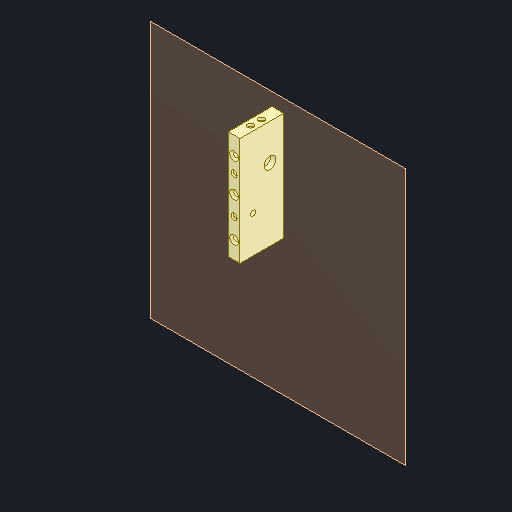
# Autodesk Inventor part: middle_gear_holder
Saved by Autodesk Inventor 2023 (Build 270158000, 158)
## iProperties
Created: 2024-04-23
Part Number: middle_gear_holder
Material: Nylon 6/6
Document SubType Name: Modeling
Designer: szymo
Density: 1.13 g/cm^3
Appearance: Nylon 6
Mass: 25.6721 g
Surface Area: 95.1123 cm^2
Volume: 22.7187 cm^3
Author: szymo
Autodesk Inventor part; units mm, degrees
ref_plane "YZ Plane" through (0, 0, 0) normal (1, 0, 0) x (0, 1, 0)
ref_plane "XZ Plane" through (0, 0, 0) normal (0, 1, 0) x (-1, 0, 0)
ref_plane "Work Plane1" through (0, 0, 0) normal (0, 0, 1) x (1, 0, 0)
ref_plane "Work Plane2" through (-89, -40.3889, 33.5) normal (0, 0, 1) x (1, 0, 0)
sketch "Sketch1" plane through (0, 0, 0) normal (0, 0, 1) x (1, 0, 0)
  line L0 (23.5, 88.5) -> (-23.5, 88.5) projected
  line L1 (-23.5, 88.5) -> (-23.5, 36.5) projected
  line L2 (-26.5, 33.5) -> (-89, 33.5) projected
  line L3 (-89, 33.5) -> (-89, -72.5) projected
  line L4 (-89, -72.5) -> (-77, -72.5) projected
  line L5 (-74, -75.5) -> (-74, -93.5) projected
  line L6 (-74, -93.5) -> (74, -93.5) projected
  line L7 (74, -93.5) -> (74, -75.5) projected
  line L8 (77, -72.5) -> (89, -72.5) projected
  line L9 (89, -72.5) -> (89, 33.5) projected
  line L10 (89, 33.5) -> (26.5, 33.5) projected
  line L11 (23.5, 36.5) -> (23.5, 88.5) projected
  line L12 (-4.5, 81.5) -> (-4.5, 36.5) projected
  line L13 (-7.5, 33.5) -> (-13.5, 33.5) projected
  line L14 (-16.5, 36.5) -> (-16.5, 81.5) projected
  line L15 (7.5, 84.5) -> (13.5, 84.5) projected
  line L16 (16.5, 81.5) -> (16.5, 36.5) projected
  line L17 (13.5, 33.5) -> (7.5, 33.5) projected
  line L18 (4.5, 36.5) -> (4.5, 81.5) projected
  line L19 (-13.5, 84.5) -> (-7.5, 84.5) projected
  line L20 (-4.5, 88.5) -> (4.5, 88.5)
  line L21 (4.5, 88.5) -> (4.5, 5.75)
  line L22 (4.5, 5.75) -> (-4.5, 5.75)
  line L23 (-4.5, 5.75) -> (-4.5, 88.5)
  line L24 (-32.2, 4.75) -> (-59.9, 4.75)
  arc A0 (13.5, 33.5) -> (16.5, 36.5) centre (13.5, 36.5) ccw projected
  arc A1 (4.5, 36.5) -> (7.5, 33.5) centre (7.5, 36.5) ccw projected
  arc A2 (7.5, 84.5) -> (4.5, 81.5) centre (7.5, 81.5) ccw projected
  arc A3 (16.5, 81.5) -> (13.5, 84.5) centre (13.5, 81.5) ccw projected
  arc A4 (-4.5, 81.5) -> (-7.5, 84.5) centre (-7.5, 81.5) ccw projected
  arc A5 (-7.5, 33.5) -> (-4.5, 36.5) centre (-7.5, 36.5) ccw projected
  arc A6 (-16.5, 36.5) -> (-13.5, 33.5) centre (-13.5, 36.5) ccw projected
  arc A7 (-13.5, 84.5) -> (-16.5, 81.5) centre (-13.5, 81.5) ccw projected
  arc A8 (-26.5, 33.5) -> (-23.5, 36.5) centre (-26.5, 36.5) ccw projected
  arc A9 (-74, -75.5) -> (-77, -72.5) centre (-77, -75.5) ccw projected
  arc A10 (77, -72.5) -> (74, -75.5) centre (77, -75.5) ccw projected
  arc A11 (23.5, 36.5) -> (26.5, 33.5) centre (26.5, 36.5) ccw projected
  circle A12 centre (21.5, -85.5) radius 1.8 projected
  circle A13 centre (-64.5, -85.5) radius 1.8 projected
  circle A14 centre (83.4, -16.3889) radius 1.8 projected
  circle A15 centre (-83.4, -19.2889) radius 1.8 projected
  circle A16 centre (-21.5, -85.5) radius 1.8 projected
  circle A17 centre (64.5, -85.5) radius 1.8 projected
  circle A18 centre (39.125, 4.3375) radius 1.0065 projected
  circle A19 centre (-72.95, 4.275) radius 1.0065 projected
  circle A20 centre (39.125, 25.9125) radius 1.0065 projected
  circle A21 centre (72.95, 12.275) radius 1.0065 projected
  circle A22 centre (86, 30.5) radius 1.0065 projected
  circle A23 centre (-86, 30.5) radius 1.0065 projected
  circle A24 centre (-39.125, 12.3375) radius 1.0065 projected
  circle A25 centre (-72.95, 25.975) radius 1.0065 projected
  circle A26 centre (-72.95, 12.275) radius 1.0065 projected
  circle A27 centre (-39.125, 25.9125) radius 1.0065 projected
  circle A28 centre (-86, 7.75) radius 1.0065 projected
  circle A29 centre (86, 7.75) radius 1.0065 projected
  circle A30 centre (72.95, 25.975) radius 1.0065 projected
  circle A31 centre (39.125, 12.3375) radius 1.0065 projected
  circle A32 centre (-39.125, 4.3375) radius 1.0065 projected
  circle A33 centre (72.95, 4.275) radius 1.0065 projected
  circle A34 centre (78, -67.1725) radius 1.2295 projected
  circle A35 centre (-24.1, -73.1) radius 1.2295 projected
  circle A36 centre (24.1, -24.9) radius 1.2295 projected
  circle A37 centre (-42.4984, -44.6666) radius 1.2295 projected
  circle A38 centre (-79, -42.3889) radius 1.2295 projected
  circle A39 centre (-19.5, 28.875) radius 1.2295 projected
  circle A40 centre (19.5, 9.55) radius 1.2295 projected
  circle A41 centre (19.5, 47.3) radius 1.2295 projected
  circle A42 centre (-19.5, 47.3) radius 1.2295 projected
  circle A43 centre (0, 74.7) radius 1.2295 projected
  circle A44 centre (-19.4231, 74.8077) radius 1.2295 projected
  circle A45 centre (19.5, 74.7) radius 1.2295 projected
  circle A46 centre (0, 49.05) radius 1.2295 projected
  circle A47 centre (19.5, 28.875) radius 1.2295 projected
  circle A48 centre (0, 19.125) radius 1.2295 projected
  circle A49 centre (-19.5, 9.55) radius 1.2295 projected
  circle A50 centre (-78, -67.1725) radius 1.2295 projected
  circle A51 centre (-24.1, -24.9) radius 1.2295 projected
  circle A52 centre (24.1, -73.1) radius 1.2295 projected
  circle A53 centre (42.5, -44.6649) radius 1.2295 projected
  circle A54 centre (79, -42.3889) radius 1.2295 projected
  line L25 (74, -12.9454) -> (74, -38.6649) projected
  line L26 (32.5736, -41.3399) -> (10.2484, -66.6122) projected
  line L27 (40.7223, -24.1882) -> (40.7223, -2.7315) projected
  line L28 (15.0791, 0.2685) -> (31.7223, 0.2685) projected
  line L29 (-68.7516, -10.9592) -> (-46.0313, -36.6788) projected
  line L30 (-74, -38.6649) -> (-74, -12.9454) projected
  line L31 (43.7223, 0.2685) -> (62.6769, 0.2685) projected
  line L32 (-40.7223, -2.7315) -> (-40.7223, -24.1882) projected
  line L33 (-45.9707, -26.1743) -> (-64.9252, -4.7177) projected
  line L34 (46.0313, -36.6788) -> (68.7516, -10.9592) projected
  line L35 (-62.6769, 0.2685) -> (-43.7223, 0.2685) projected
  line L36 (34.7223, -2.7315) -> (34.7223, -24.9078) projected
  line L37 (29.5555, -26.9826) -> (10.5667, -7.1519) projected
  line L38 (-31.598, -53.0174) -> (-25.9833, -59.3733) projected
  line L39 (-10.5667, -7.1519) -> (-29.5555, -26.9826) projected
  line L40 (-34.7223, -24.9078) -> (-34.7223, -2.7315) projected
  line L41 (-31.7223, 0.2685) -> (-15.0791, 0.2685) projected
  line L42 (25.9833, -59.3733) -> (31.598, -53.0174) projected
  line L43 (64.9252, -4.7177) -> (45.9707, -26.1743) projected
  line L44 (-10.2484, -66.6122) -> (-32.5736, -41.3399) projected
  line L45 (-32.4921, -37.2789) -> (-10.1668, -13.9638) projected
  line L46 (10.1668, -13.9638) -> (32.4921, -37.2789) projected
  line L47 (29.5955, -81.1563) -> (25.3044, -62.0157) projected
  arc A55 (25.9833, -59.3733) -> (25.3044, -62.0157) centre (28.2317, -61.3594) ccw projected
  line L48 (43.9754, -47.6649) -> (68.9203, -47.6649) projected
  arc A56 (71.5475, -52.1134) -> (68.9203, -47.6649) centre (68.9203, -50.6649) ccw projected
  line L49 (71.5475, -52.1134) -> (58.4661, -75.8408) projected
  line L50 (46.5943, -83.5) -> (32.5229, -83.5) projected
  arc A57 (29.5955, -81.1563) -> (32.5229, -83.5) centre (32.5229, -80.5) ccw projected
  line L51 (-5, -16.0387) -> (-5, -64.6261) projected
  arc A58 (-10.2484, -66.6122) -> (-5, -64.6261) centre (-8, -64.6261) ccw projected
  arc A59 (-32.4921, -37.2789) -> (-32.5736, -41.3399) centre (-30.3253, -39.3537) ccw projected
  arc A60 (-5, -16.0387) -> (-10.1668, -13.9638) centre (-8, -16.0387) ccw projected
  arc A61 (-40.7223, -2.7315) -> (-43.7223, 0.2685) centre (-43.7223, -2.7315) ccw projected
  arc A62 (-45.9707, -26.1743) -> (-40.7223, -24.1882) centre (-43.7223, -24.1882) ccw projected
  arc A63 (-62.6769, 0.2685) -> (-64.9252, -4.7177) centre (-62.6769, -2.7315) ccw projected
  arc A64 (-25.3044, -62.0157) -> (-25.9833, -59.3733) centre (-28.2317, -61.3594) ccw projected
  line L52 (-25.3044, -62.0157) -> (-29.5955, -81.1563) projected
  arc A65 (-32.5229, -83.5) -> (-29.5955, -81.1563) centre (-32.5229, -80.5) ccw projected
  line L53 (-32.5229, -83.5) -> (-46.5943, -83.5) projected
  line L54 (-58.4661, -75.8408) -> (-71.5475, -52.1134) projected
  arc A66 (-68.9203, -47.6649) -> (-71.5475, -52.1134) centre (-68.9203, -50.6649) ccw projected
  line L55 (-68.9203, -47.6649) -> (-43.9754, -47.6649) projected
  line L56 (-49.775, 11.125) -> (-62.3, 11.125) projected
  arc A67 (-62.3, 27.125) -> (-62.3, 11.125) centre (-62.3, 19.125) ccw projected
  line L57 (-62.3, 27.125) -> (-49.775, 27.125) projected
  arc A68 (-49.775, 11.125) -> (-49.775, 27.125) centre (-49.775, 19.125) ccw projected
  arc A69 (-31.7223, 0.2685) -> (-34.7223, -2.7315) centre (-31.7223, -2.7315) ccw projected
  arc A70 (-12.9578, -0.6102) -> (-15.0791, 0.2685) centre (-15.0791, -2.7315) ccw projected
  line L58 (-12.9578, -0.6102) -> (-10.6122, -2.9558) projected
  arc A71 (-10.5667, -7.1519) -> (-10.6122, -2.9558) centre (-12.7335, -5.0771) ccw projected
  arc A72 (-34.7223, -24.9078) -> (-29.5555, -26.9826) centre (-31.7223, -24.9078) ccw projected
  arc A73 (71, -41.6649) -> (74, -38.6649) centre (71, -38.6649) ccw projected
  line L59 (71, -41.6649) -> (48.2797, -41.6649) projected
  arc A74 (46.0313, -36.6788) -> (48.2797, -41.6649) centre (48.2797, -38.6649) ccw projected
  arc A75 (74, -12.9454) -> (68.7516, -10.9592) centre (71, -12.9454) ccw projected
  arc A76 (40.7223, -24.1882) -> (45.9707, -26.1743) centre (43.7223, -24.1882) ccw projected
  arc A77 (43.7223, 0.2685) -> (40.7223, -2.7315) centre (43.7223, -2.7315) ccw projected
  arc A78 (64.9252, -4.7177) -> (62.6769, 0.2685) centre (62.6769, -2.7315) ccw projected
  arc A79 (5, -64.6261) -> (10.2484, -66.6122) centre (8, -64.6261) ccw projected
  line L60 (5, -64.6261) -> (5, -16.0387) projected
  arc A80 (10.1668, -13.9638) -> (5, -16.0387) centre (8, -16.0387) ccw projected
  arc A81 (32.5736, -41.3399) -> (32.4921, -37.2789) centre (30.3253, -39.3537) ccw projected
  arc A82 (29.5555, -26.9826) -> (34.7223, -24.9078) centre (31.7223, -24.9078) ccw projected
  arc A83 (10.6122, -2.9558) -> (10.5667, -7.1519) centre (12.7335, -5.0771) ccw projected
  line L61 (10.6122, -2.9558) -> (12.9578, -0.6102) projected
  arc A84 (15.0791, 0.2685) -> (12.9578, -0.6102) centre (15.0791, -2.7315) ccw projected
  arc A85 (34.7223, -2.7315) -> (31.7223, 0.2685) centre (31.7223, -2.7315) ccw projected
  arc A86 (-48.2797, -41.6649) -> (-46.0313, -36.6788) centre (-48.2797, -38.6649) ccw projected
  line L62 (-48.2797, -41.6649) -> (-71, -41.6649) projected
  arc A87 (-74, -38.6649) -> (-71, -41.6649) centre (-71, -38.6649) ccw projected
  arc A88 (-68.7516, -10.9592) -> (-74, -12.9454) centre (-71, -12.9454) ccw projected
  line L63 (49.775, 27.125) -> (62.3, 27.125) projected
  arc A89 (62.3, 11.125) -> (62.3, 27.125) centre (62.3, 19.125) ccw projected
  line L64 (62.3, 11.125) -> (49.775, 11.125) projected
  arc A90 (49.775, 27.125) -> (49.775, 11.125) centre (49.775, 19.125) ccw projected
  arc A91 (53.1556, -75.734) -> (58.4661, -75.8408) centre (55.8389, -74.3924) ccw projected
  line L65 (53.1556, -75.734) -> (41.2921, -52.0066) projected
  arc A92 (43.9754, -47.6649) -> (41.2921, -52.0066) centre (43.9754, -50.6649) ccw projected
  arc A93 (36.5297, -53.662) -> (31.598, -53.0174) centre (33.8464, -55.0036) ccw projected
  line L66 (36.5297, -53.662) -> (49.2776, -79.1584) projected
  arc A94 (46.5943, -83.5) -> (49.2776, -79.1584) centre (46.5943, -80.5) ccw projected
  arc A95 (-49.2776, -79.1584) -> (-46.5943, -83.5) centre (-46.5943, -80.5) ccw projected
  line L67 (-49.2776, -79.1584) -> (-36.5297, -53.662) projected
  arc A96 (-31.598, -53.0174) -> (-36.5297, -53.662) centre (-33.8464, -55.0036) ccw projected
  arc A97 (-41.2921, -52.0066) -> (-43.9754, -47.6649) centre (-43.9754, -50.6649) ccw projected
  line L68 (-41.2921, -52.0066) -> (-53.1556, -75.734) projected
  arc A98 (-58.4661, -75.8408) -> (-53.1556, -75.734) centre (-55.8389, -74.3924) ccw projected
  point P0 (0, 0)
  point P1 (-4.5, 81.5)
  point P2 (-4.5, 36.5)
  point P3 (7.5, 81.5)
  point P4 (13.5, 81.5)
  point P5 (-7.5, 81.5)
  point P6 (-13.5, 81.5)
  point P7 (-29, -78.5)
  point P8 (-57, -78.5)
  point P9 (29, -78.5)
  point P10 (57, -78.5)
  dimension "d41" = 1
  constraints: 10 end point, 2 collinear, 2 horizontal, 2 parallel, 1 perpendicular, 1 point on line, 2 other
  measures "d41" distance between parallel lines of L22 L24
extrude "Extrusion1" add sketch "Sketch1" along normal up to surface (33.5 mm away) contours L21 L18 L22 L23 L12 L0 | A43 | A46 | A48
sketch "Sketch2" plane through (4.5, 5.75, 0) normal (1, 0, 0) x (0, 0, -1)
  circle A0 centre (-23.4363, 28.1825) radius 2 projected
  point P0 (0, -5.75)
extrude "Extrusion2" cut sketch "Sketch2" against normal blind 10
sketch "Sketch3" plane through (4.5, 5.75, 0) normal (1, 0, 0) x (0, 0, -1)
  circle A0 centre (-10.5, 55.25) radius 4.5 projected
  point P0 (0, -5.75)
extrude "Extrusion3" cut sketch "Sketch3" against normal blind 4
sketch "Sketch4" plane through (-4.5, 5.75, 0) normal (-1, 0, 0) x (0, 0, 1)
  circle A0 centre (10.5, 55.25) radius 4.5 projected
  point P0 (0, -5.75)
extrude "Extrusion4" cut sketch "Sketch4" against normal blind 4
sketch "Sketch5" plane through (-4.5, 5.75, 33.5) normal (0, 0, 1) x (1, 0, 0)
  line L0 (5, 59.75) -> (5, 50.75) projected
  line L1 (4, 50.75) -> (4, 59.75) projected
  line L2 (9, 26.1825) -> (0, 26.1825) projected
  line L3 (9, 30.1825) -> (0, 30.1825) projected
  line L4 (17, 78.15) -> (-8, 78.15)
  line L5 (-8, 35.85) -> (17, 35.85)
  line L6 (9, 82.75) -> (9, 0) projected
  line L7 (0, 50.75) -> (0, 59.75) projected
  line L8 (9, 35.85) -> (0, 35.85)
  line L9 (0, 35.85) -> (0, 50.75)
  line L10 (0, 50.75) -> (9, 50.75)
  line L11 (9, 50.75) -> (9, 35.85)
  line L12 (0, 0) -> (0, 82.75) projected
  line L13 (9, 78.15) -> (0, 78.15)
  line L14 (0, 78.15) -> (0, 59.75)
  line L15 (0, 59.75) -> (9, 59.75)
  line L16 (9, 59.75) -> (9, 78.15)
  line L17 (-18, 6.625) -> (-18, 20.125) projected
  line L18 (-18, 13.375) -> (27, 13.375)
  line L19 (9, 35.85) -> (0, 50.75)
  line L20 (9, 59.75) -> (9, 50.75) projected
  line L21 (0, 35.85) -> (9, 50.75)
  line L22 (9, 59.75) -> (0, 78.15)
  line L23 (0, 59.75) -> (9, 78.15)
  point P0 (4.5, -5.75)
  point P1 (4.5, 13.375)
  point P2 (4.5, 43.3)
  point P3 (4.5, 68.95)
  dimension "d9" = 4.5
  dimension "d10" = 4.5
  constraints: 30 end point, 5 horizontal, 5 point on line, 4 midpoint, 4 parallel, 2 perpendicular, 4 other
  measures "d9" distance from line of L6 point (4.5, 13.375)
  measures "d10" distance from line of point (4.5, 13.375) L12
hole "Hole1" at (0, 19.125, 33.5) at (0, 49.05, 33.5) at (0, 74.7, 33.5) direction (0, 0, -1) diameter 3.6 end through all countersink diameter 6.6 countersink angle 90 clearance for "Countersunk Flat Head Screw ISO 2009/7046" size "M3" standard "ISO"
sketch "Sketch6" plane through (-4.5, 5.75, 0) normal (0, -1, 0) x (1, 0, 0)
  line L0 (9, 33.5) -> (0, 33.5) projected
  line L1 (0, 0) -> (0, 33.5) projected
  line L2 (0, 0) -> (9, 0) projected
  line L3 (9, 0) -> (9, 33.5) projected
  line L4 (0, 16.75) -> (9, 16.75)
  line L5 (9, 16.75) -> (0, 33.5)
  line L6 (9, 33.5) -> (0, 16.75)
  line L7 (0, 16.75) -> (9, 0)
  line L8 (9, 16.75) -> (0, 0)
  point P0 (4.5, 0)
  point P1 (4.5, 8.375)
  point P2 (4.5, 25.125)
  constraints: 10 end point, 4 midpoint, 2 parallel
hole "Hole2" at (0, 5.75, 8.375) at (0, 5.75, 25.125) direction (0, 1, 0) diameter 4 depth 6.6 counterbore diameter 5 counterbore depth 2
sketch "Sketch7" plane through (-4.5, 88.5, 0) normal (0, 1, 0) x (1, 0, 0)
  line L0 (0, -33.5) -> (9, -33.5) projected
  line L1 (0, -33.5) -> (9, -33.5) projected
  line L2 (9, 0) -> (9, -33.5) projected
  line L3 (9, 0) -> (0, 0) projected
  line L4 (0, 0) -> (0, -33.5) projected
  line L5 (-8, -1.4) -> (-8, -6.6) projected
  line L6 (-8, -32.1) -> (-8, -26.9) projected
  line L7 (17, -32.1) -> (17, -26.9) projected
  line L8 (17, -1.4) -> (17, -6.6) projected
  line L9 (17, -32.1) -> (-8, -32.1)
  line L10 (-8, -32.1) -> (-8, -26.9)
  line L11 (-8, -26.9) -> (17, -26.9)
  line L12 (17, -26.9) -> (17, -32.1)
  line L13 (-8, -6.6) -> (17, -6.6)
  line L14 (17, -6.6) -> (17, -1.4)
  line L15 (17, -1.4) -> (-8, -1.4)
  line L16 (-8, -1.4) -> (-8, -6.6)
  line L17 (17, -6.6) -> (-8, -6.6)
  line L18 (-8, -6.6) -> (-8, -8.6)
  line L19 (-8, -8.6) -> (17, -8.6)
  line L20 (17, -8.6) -> (17, -6.6)
  line L21 (-8, -26.9) -> (17, -26.9)
  line L22 (17, -26.9) -> (17, -24.9)
  line L23 (17, -24.9) -> (-8, -24.9)
  line L24 (-8, -24.9) -> (-8, -26.9)
  line L25 (9, 0) -> (9, -33.5) projected
  line L26 (9, -16.75) -> (0, -16.75)
  line L27 (0, 0) -> (0, -33.5) projected
  line L28 (9, -24.9) -> (0, -16.75)
  line L29 (9, -8.6) -> (0, -16.75)
  line L30 (0, -8.6) -> (9, -16.75)
  line L31 (9, -16.75) -> (0, -24.9)
  point P0 (4.5, 0)
  point P1 (4.5, -20.825)
  point P2 (4.5, -12.675)
  dimension "d25" = 2
  dimension "d26" = 2
  constraints: 42 end point, 10 point on line, 8 parallel, 5 midpoint, 4 horizontal, 4 perpendicular
  measures "d25" distance of L18.end L17.end
  measures "d26" distance of L22.end L21.end
hole "Hole3" at (0, 88.5, 20.825) at (0, 88.5, 12.675) direction (0, -1, 0) diameter 4 depth 6.5 counterbore diameter 4.6 counterbore depth 2
sketch "Sketch8" plane through (-4.5, 5.75, 33.5) normal (0, 0, 1) x (1, 0, 0)
  line L0 (26, 27.2497) -> (-17, 27.2497)
  line L1 (26, 31.2497) -> (-17, 31.2497)
  line L2 (4, 52.75) -> (-1, 52.75)
  line L3 (4, 61.75) -> (-1, 61.75)
  line L4 (10, 61.75) -> (5, 61.75)
  line L5 (9, 50.75) -> (5, 50.75) projected
  line L6 (0, 0) -> (0, 82.75) projected
  line L7 (9, 52.75) -> (0, 52.75)
  line L8 (0, 52.75) -> (0, 61.75)
  line L9 (0, 61.75) -> (9, 61.75)
  line L10 (9, 61.75) -> (9, 50.75)
  line L11 (9, 26.1825) -> (0, 26.1825) projected
  line L12 (0, 31.2497) -> (9, 31.2497)
  line L13 (9, 31.2497) -> (9, 26.1825)
  line L14 (9, 26.1825) -> (0, 26.1825)
  line L15 (0, 26.1825) -> (0, 31.2497)
  line L16 (9, 26.1825) -> (0, 31.2497)
  line L17 (0, 26.1825) -> (9, 31.2497)
  line L18 (10, 51.75) -> (0, 61.75)
  line L19 (0, 52.75) -> (9, 61.75)
  point P0 (4.5, -5.75)
  point P1 (4.5, 28.7161)
  point P2 (4.5, 57.25)
  constraints: 34 end point, 7 horizontal, 6 point on line, 4 parallel, 3 perpendicular, 2 midpoint, 10 other
hole "Hole4" at (0, 34.4661, 33.5) at (0, 63, 33.5) direction (0, 0, -1) diameter 4 depth 6 counterbore diameter 4.6 counterbore depth 1.5
equation "\"d9\" = d10"
body "Solid1"
